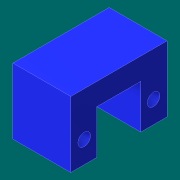
# Autodesk Inventor part: mppcMount
Saved by Autodesk Inventor 2016 (Build 200138000, 138)
## iProperties
Created: 2016-02-18
Part Number: mppcMount
Material: ABS Plastic
Document SubType Name: Modeling
Designer: Sawaiz
Density: 1.06 g/cm^3
Appearance: Blue - Wall Paint - Glossy
Author: Sawaiz
Autodesk Inventor part; units mm, degrees
ref_plane "YZ Plane" through (0, 0, 0) normal (1, 0, 0) x (0, 1, 0)
ref_plane "XZ Plane" through (0, 0, 0) normal (0, 1, 0) x (-1, 0, 0)
ref_plane "XY Plane" through (0, 0, 0) normal (0, 0, 1) x (1, 0, 0)
sketch "Sketch1" plane through (0, 0, 0) normal (0, 1, 0) x (-1, 0, 0)
  line L0 (-12.5, -11.4) -> (-5.7, -11.4)
  line L1 (-5.7, -11.4) -> (-5.7, 0)
  line L2 (-5.7, 0) -> (5.7, 0)
  line L3 (5.7, 0) -> (5.7, -11.4)
  line L4 (5.7, -11.4) -> (12.5, -11.4)
  line L5 (12.5, -11.4) -> (12.5, 5.7)
  line L6 (12.5, 5.7) -> (-12.5, 5.7)
  line L7 (-12.5, 5.7) -> (-12.5, -11.4)
  line L8 (0, 0) -> (0, 5.7) construction
  dimension "d0" = 11.4
  dimension "d1" = 11.4
  dimension "d4" = 5.7
  dimension "d17" = 25
  constraints: 18 end point, 6 perpendicular, 2 midpoint, 2 point on line, 1 coincident, 1 horizontal, 1 vertical
  measures "d0" distance of L1.end L2.end
  measures "d1" distance of L0.end L1.end
  measures "d4" distance between parallel lines of L6 L2
  measures "d17" distance between parallel lines of L5 L7
extrude "Extrusion1" add sketch "Sketch1" along normal blind 15
sketch "Sketch2" plane through (0, 15, 0) normal (0, 1, 0) x (1, 0, 0)
  line L0 (12.5, 11.4) -> (5.7, 11.4) projected
  line L1 (5.7, 11.4) -> (5.7, 0) projected
  line L2 (5.7, 0) -> (-5.7, 0) projected
  line L3 (-5.7, 0) -> (-5.7, 11.4) projected
  line L4 (-5.7, 11.4) -> (-12.5, 11.4) projected
  line L5 (-12.5, 11.4) -> (-12.5, -5.7) projected
  line L6 (-12.5, -5.7) -> (12.5, -5.7) projected
  line L7 (12.5, -5.7) -> (12.5, 11.4) projected
  line L8 (12.5, -5.7) -> (12.5, 11.4) construction
  line L9 (-5.7, 11.4) -> (-12.5, 11.4) construction
  line L10 (-12.5, 11.4) -> (-12.5, -5.7) construction
  line L11 (9, 5.7) -> (-9, 5.7) construction
  line L12 (0, 5.7) -> (0, 0) construction
  dimension "d14" = 18
  dimension "d15" = 5.7
  dimension "d16" = 11.4
  constraints: 4 end point, 2 coincident, 1 horizontal, 1 midpoint, 1 perpendicular
  measures "d14" distance of point (-9, 5.7) point (9, 5.7)
  measures "d15" distance between parallel lines of L2 L11
  measures "d16" distance of L0.end L1.end
hole "Hole1" at (9, 15, -5.7) at (-9, 15, -5.7) direction (0, -1, 0) diameter 3.264 depth 8 tip angle 118 clearance for "Oval Head Machine Screw" size "#4" standard "Ansi Unified Screw Threads"
equation "\"d0\" = 2 * silveringThickness + ScintillatorWidth + 2 * rubberizedCoating"
equation "\"d1\" = 2 * silveringThickness + ScintillatorWidth + 2 * rubberizedCoating"
equation "\"d4\" = rubberizedCoating + 0.5 * ScintillatorWidth + silveringThickness"
equation "\"d14\" = 2 * MountingScrewOffsett"
equation "\"d15\" = 0.5 * d16"
equation "\"OpticalFiberClearence\" = 0.1"
equation "\"ScintillatorEdgeClearence\" = 3"
equation "\"ShallowTrackDepth\" = 1.2"
equation "\"DeepTrackDepth\" = 5.6"
equation "\"FiberEdgeOffsett\" = 5"
equation "\"LoopLargeTrackRatio\" = 1.1"
equation "\"FiberSensorClerence\" = 0.5"
equation "\"MountingScrewOffsett\" = 9"
equation "\"silveringThickness\" = 0.2"
equation "\"rubberizedCoating\" = 0.5"
equation "\"ScintillatorWidth\" = 10"
body "Solid1"
